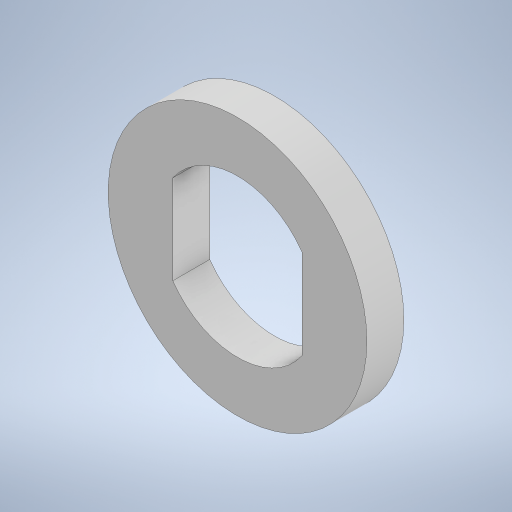
# Autodesk Inventor part: ANT_SPACER
Saved by Autodesk Inventor 2024 (Build 280153000, 153)
## iProperties
Created: 2026-02-20
Part Number: ANT_SPACER
Material: Типовые
Document SubType Name: Modeling
Designer: fm
Density: 1 g/cm^3
Appearance: По умолчанию
Author: fm
Autodesk Inventor part; units mm, degrees
ref_plane "YZ Plane" through (0, 0, 0) normal (1, 0, 0) x (0, 1, 0)
ref_plane "XZ Plane" through (0, 0, 0) normal (0, 1, 0) x (-1, 0, 0)
ref_plane "XY Plane" through (0, 0, 0) normal (0, 0, 1) x (1, 0, 0)
sketch "Эскиз1" plane through (0, 0, 0) normal (0, 0, 1) x (1, 0, 0)
  circle A0 centre (0, 0) radius 4.25
  circle A1 centre (0, 0) radius 7
  line L0 (-3.5, 0) -> (3.5, 0)
  line L1 (-3.5, 2.4109) -> (-3.5, -2.4109)
  line L2 (3.5, 2.4109) -> (3.5, -2.4109)
  dimension "d0" = 8.5
  dimension "d1" = 14
  dimension "d2" = 7
  constraints: 6 end point, 3 coincident, 3 midpoint, 2 centre point, 2 point on circle, 2 vertical, 1 horizontal
  measures "d0" diameter of A0
  measures "d1" diameter of A1
  measures "d2" distance of L0.end L0.start
extrude "Выдавливание1" add sketch "Эскиз1" along normal blind 2 contours A0 L2 | L1 A0 | A1
